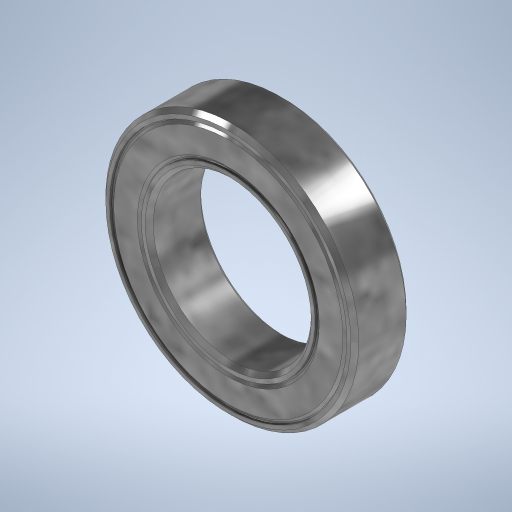
# Autodesk Inventor part: 6203베어링
Saved by Autodesk Inventor 2023 (Build 270158000, 158)
## iProperties
Created: 2022-06-08
Part Number: 6203베어링
Material: 일반
Document SubType Name: Modeling
Designer: fly01
Density: 1 g/cm^3
Appearance: 기본값
Author: fly01
Autodesk Inventor part; units mm, degrees
ref_plane "YZ Plane" through (0, 0, 0) normal (1, 0, 0) x (0, 1, 0)
ref_plane "XZ Plane" through (0, 0, 0) normal (0, 1, 0) x (-1, 0, 0)
ref_plane "XY Plane" through (0, 0, 0) normal (0, 0, 1) x (1, 0, 0)
sketch "스케치1" plane through (0, 0, 0) normal (0, 0, 1) x (1, 0, 0)
  circle A0 centre (0, 0) radius 10
  circle A1 centre (0, 0) radius 16
  dimension "d0" = 20
  dimension "d1" = 32
  constraints: 2 centre point, 2 coincident
  measures "d0" diameter of A0
  measures "d1" diameter of A1
extrude "돌출1" add sketch "스케치1" along normal mid plane 7
chamfer "모따기1" distance 0.5 angle 45 4 edges at (-16, 0, 3.5) (-16, 0, -3.5) (-10, 0, 3.5) (-10, 0, -3.5)
sketch "스케치2" plane through (0, 0, 0) normal (0, 1, 0) x (-1, 0, 0)
  line L0 (-15.5, 3.5) -> (15.5, 3.5) projected
  line L1 (15, 3.5) -> (15, 3.2414)
  line L2 (14.8293, 3.1707) -> (14.5, 3.5)
  line L3 (16, 0) -> (10, 0)
  line L4 (10, 3) -> (10, -3) projected
  arc A0 (14.8293, 3.1707) -> (15, 3.2414) centre (14.9, 3.2414) ccw
  line L5 (13, 0) -> (13, 1.7292)
  line L6 (11, 3.5) -> (11, 3.2414)
  line L7 (11.1707, 3.1707) -> (11.5, 3.5)
  arc A1 (11, 3.2414) -> (11.1707, 3.1707) centre (11.1, 3.2414) ccw
  line L8 (15, -3.5) -> (15, -3.2414)
  line L9 (14.8293, -3.1707) -> (14.5, -3.5)
  arc A2 (15, -3.2414) -> (14.8293, -3.1707) centre (14.9, -3.2414) ccw
  line L10 (11, -3.5) -> (11, -3.2414)
  line L11 (11.1707, -3.1707) -> (11.5, -3.5)
  arc A3 (11.1707, -3.1707) -> (11, -3.2414) centre (11.1, -3.2414) ccw
  line L12 (0, 0) -> (0, -13.1586)
  line L13 (15.5, -3.5) -> (-15.5, -3.5) projected
  line L14 (16, -3) -> (16, 3) projected
  point P0 (15, 3)
  point P1 (10.5, 3.5)
  point P2 (11, 3)
  point P3 (15, -3)
  point P4 (10.5, -3.5)
  point P5 (11, -3)
  dimension "d7" = 0.5
  dimension "d8" = 0.5
  dimension "d9" = 0.5
  dimension "d10" = 0.1
  constraints: 22 end point, 21 symmetric about line, 10 point on line, 8 point on circle, 4 centre point, 3 midpoint, 3 vertical, 2 tangent, 3 other
  measures "d7" distance of L0.end L1.start
  measures "d8" distance of L1.start point (15, 3)
  measures "d9" distance of L1.start L2.end
  measures "d10" radius of A0
revolve "회전1" cut sketch "스케치2" angle 360 about axis through (0, 0, 0) along (0, 0, -1)
